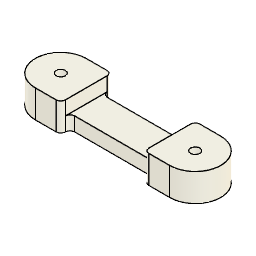
(Unsaved) (Autodesk Fusion 360 design; units mm, degrees)
Autodesk Fusion 360 part; units mm, degrees
sketch "Sketch1" plane through (0, 0, 0) normal (0, 0, 1) x (1, 0, 0)
  line L0 (-74, -11) -> (-16, -11)
  line L1 (-16, 11) -> (-74, 11)
  arc A0 (-74, 11) -> (-74, -11) centre (-74, 0) ccw
  arc A1 (-16, -11) -> (-16, 11) centre (-16, 0) ccw
  circle A2 centre (-74, 0) radius 2
  circle A3 centre (-16, 0) radius 2
  line L2 (-63, 11) -> (-63, -11)
  line L3 (-27, 11) -> (-27, -11)
  line L4 (-63, 7) -> (-27, 7)
  line L5 (-63, -7) -> (-27, -7)
  dimension "d1" = 4
  dimension "d2" = 4
  constraint concentric A0 A2
  constraint concentric A1 A3
  constraint coincident L1 L2.start
  constraint coincident L0 L2.end
  constraint coincident L1 L3.start
  constraint coincident L0 L3.end
  constraint perpendicular L0 L3
  constraint coincident L2 L4.start
  constraint coincident L2 L5.start
  constraint coincident L3 L5.end
  constraint perpendicular L3 L5
  measures "d1" diameter of A2
  measures "d2" diameter of A3
extrude "Extrude1" add sketch "Sketch1" along normal blind 12 contours L0 L1 A0 L2 | L0 L1 A1 L3 makes body 1 at (-66, 0, 0) makes body 2 at (-24, 0, 0)
extrude "Extrude2" add sketch "Sketch1" along normal blind 6 contours L2 L3 L4 L5 bodies 1 2
chamfer "Chamfer1" distance 1.5 angle 45 2 edges at (-75.8647, 0.7232, 0) (-17.8647, 0.7232, 0) on bodies 1
fillet "Fillet1" radius 2 4 edges at (-63, -7, 3) (-27, -7, 3) (-27, 7, 3) (-63, 7, 3) on bodies 1
fillet "Fillet2" radius 2 4 edges at (-63, 11, 6) (-27, 11, 6) (-27, -11, 6) (-63, -11, 6) on bodies 1
